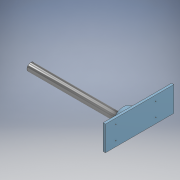
# Autodesk Inventor part: DecAxis
Saved by Autodesk Inventor 2022 (Build 260153000, 153)
## iProperties
Created: 2021-05-01
Part Number: DecAxis
Material: Generic
Document SubType Name: Modeling
Designer: Mick Veldhuis
Density: 1 g/cm^3
Appearance: Default
Author: Mick Veldhuis
Autodesk Inventor part; units mm, degrees
ref_plane "YZ Plane" through (0, 0, 0) normal (1, 0, 0) x (0, 1, 0)
ref_plane "XZ Plane" through (0, 0, 0) normal (0, 1, 0) x (-1, 0, 0)
ref_plane "XY Plane" through (0, 0, 0) normal (0, 0, 1) x (1, 0, 0)
sketch "Sketch1" plane through (0, 0, 0) normal (1, 0, 0) x (0, 1, 0)
  circle A0 centre (0, 0) radius 33
  constraints: 1 centre point, 1 coincident
extrude "Extrusion1" add sketch "Sketch1" against normal blind 600
sketch "Sketch2" plane through (0, 0, 0) normal (1, 0, 0) x (0, 0, -1)
  circle A0 centre (0, 0) radius 33
  constraints: 1 centre point, 1 coincident
extrude "Extrusion2" add sketch "Sketch2" along normal blind 198
sketch "Sketch3" plane through (198, 0, 0) normal (1, 0, 0) x (0, 0, -1)
  circle A0 centre (0, 0) radius 103
  constraints: 1 centre point, 1 coincident
extrude "Extrusion3" add sketch "Sketch3" along normal blind 36
sketch "Sketch4" plane through (234, 0, 0) normal (1, 0, 0) x (0, 0, -1)
  line L0 (-212, 107) -> (212, 107)
  line L1 (212, -107) -> (-212, -107)
  line L2 (-212, -107) -> (-212, 107)
  line L3 (-212, 107) -> (212, -107) construction
  line L4 (212, 107) -> (-212, -107) construction
  line L5 (212, 107) -> (376, 107)
  line L6 (376, 107) -> (376, -107)
  line L7 (376, -107) -> (212, -107)
  point P0 (0, 0)
  point P1 (0, 0)
  constraints: 16 end point, 2 horizontal, 2 midpoint, 2 parallel, 1 perpendicular
extrude "Extrusion4" add sketch "Sketch4" along normal blind 20
sketch "Sketch5" plane through (254, 0, 0) normal (1, 0, 0) x (0, 0, -1)
  point P0 (0, 0)
  point P1 (-124.0692, -60)
  point P2 (-124, 60)
  point P3 (220, 60)
  point P4 (220, -60)
hole "Hole1" at (254, -60, 124.0692) at (254, 60, 124) at (254, 60, -220) at (254, -60, -220) direction (-1, 0, 0) diameter 6.647 depth 20 thread size "M8x1.25" class "6H" standard "ISO Metric profile"
body "Solid1"
